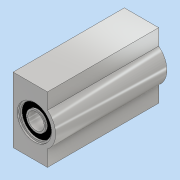
# Autodesk Inventor part: Łożysko liniowe w obudowie SMAG10UU-L
Saved by Autodesk Inventor 2018 (Build 220112000, 112)
## iProperties
Created: 2019-02-01
Part Number: Łożysko liniowe w obudowie SMAG10UU-L
Material: Ogólny
Document SubType Name: Modeling
Designer: Dawid
Density: 1 g/cm^3
Appearance: Aluminium — ciemne
Author: Dawid
Autodesk Inventor part; units mm, degrees
ref_plane "YZ Plane" through (0, 0, 0) normal (1, 0, 0) x (0, 1, 0)
ref_plane "XZ Plane" through (0, 0, 0) normal (0, 1, 0) x (-1, 0, 0)
ref_plane "XY Plane" through (0, 0, 0) normal (0, 0, 1) x (1, 0, 0)
sketch "Szkic1" plane through (0, 0, 0) normal (0, 1, 0) x (-1, 0, 0)
  line L0 (-8, 20) -> (13, 20)
  line L1 (13, 20) -> (13, -20)
  line L2 (13, -20) -> (-8, -20)
  line L3 (-13, 20) -> (13, -20) construction
  line L4 (13, 20) -> (-13, -20) construction
  line L5 (13, 0) -> (0, 0)
  circle A0 centre (0, 0) radius 5
  line L6 (13, 20) -> (-8, 20)
  arc A1 (-8, 10.247) -> (-8, -10.247) centre (0, 0) ccw
  line L7 (-8, 20) -> (-8, 10.247)
  line L8 (-8, -10.247) -> (-8, -20)
  dimension "d0" = 26
  dimension "d1" = 40
  dimension "d2" = 10
  dimension "d3" = 21
  constraints: 18 end point, 5 midpoint, 3 perpendicular, 2 centre point, 2 horizontal, 2 point on circle, 1 parallel
  measures "d0" distance of L1.end L4.end
  measures "d1" distance of L0.end L1.end
  measures "d2" diameter of A0
  measures "d3" distance of L0.start L0.end
extrude "Wyciągnięcie proste1" add sketch "Szkic1" along normal blind 68
sketch "Szkic2" plane through (0, 68, 0) normal (0, 1, 0) x (1, 0, 0)
  circle A0 centre (0, 0) radius 5 projected
  circle A1 centre (0, 0) radius 6
  circle A2 centre (0, 0) radius 10.5
  circle A3 centre (0, 0) radius 9.5
  dimension "d6" = 12
  dimension "d7" = 21
  dimension "d8" = 19
  constraints: 3 centre point, 3 coincident
  measures "d6" diameter of A1
  measures "d7" diameter of A2
  measures "d8" diameter of A3
extrude "Wyciągnięcie proste2" cut sketch "Szkic2" against normal blind 1
sketch "Szkic3" plane through (0, 68, 0) normal (0, 1, 0) x (1, 0, 0)
  circle A0 centre (0, 0) radius 6 projected
  circle A1 centre (0, 0) radius 9.5 projected
extrude "Wyciągnięcie proste3" cut sketch "Szkic3" against normal blind 2
sketch "Szkic4" plane through (0, 0, 0) normal (0, -1, 0) x (1, 0, 0)
  circle A0 centre (0, 0) radius 5
  circle A1 centre (0, 0) radius 6
  circle A2 centre (0, 0) radius 10.5
  circle A3 centre (0, 0) radius 9.5
  dimension "d13" = 12
  dimension "d14" = 21
  dimension "d15" = 19
  constraints: 4 centre point, 3 coincident
  measures "d13" diameter of A1
  measures "d14" diameter of A2
  measures "d15" diameter of A3
extrude "Wyciągnięcie proste4" cut sketch "Szkic4" against normal blind 1
sketch "Szkic5" plane through (0, 0, 0) normal (0, -1, 0) x (1, 0, 0)
  circle A0 centre (0, 0) radius 6 projected
  circle A1 centre (0, 0) radius 9.5 projected
extrude "Wyciągnięcie proste5" cut sketch "Szkic5" against normal blind 2
sketch "Szkic6" plane through (-13, 0, -20) normal (-1, 0, 0) x (0, 0, 1)
  line L0 (0, 0) -> (40, 0) projected
  line L1 (40, 0) -> (40, 68) projected
  line L2 (0, 68) -> (40, 68) projected
  line L3 (0, 0) -> (0, 68) projected
  line L4 (0, 68) -> (20, 68)
  line L5 (20, 68) -> (6, 68)
  line L6 (20, 68) -> (34, 68)
  line L7 (34, 68) -> (34, 0)
  line L8 (0, 0) -> (40, 0) projected
  line L9 (6, 68) -> (6, 0)
  line L10 (34, 68) -> (34, 34)
  line L11 (34, 34) -> (6, 34)
  line L12 (34, 34) -> (34, 57)
  line L13 (34, 57) -> (6, 57)
  line L14 (6, 34) -> (6, 11)
  line L15 (6, 11) -> (34, 11)
  point P0 (20, 0)
  dimension "d20" = 20
  dimension "d21" = 14
  dimension "d22" = 14
  dimension "d23" = 34
  dimension "d24" = 23
  dimension "d25" = 23
  constraints: 22 end point, 8 point on line, 4 perpendicular, 3 midpoint
  measures "d20" distance of L2.start L4.end
  measures "d21" distance of L4.end L5.end
  measures "d22" distance of L4.end L6.end
  measures "d23" distance of L6.end L10.end
  measures "d24" distance of L10.end L12.end
  measures "d25" distance of L11.end L14.end
hole "Otwór1" at (-13, 57, -14) at (-13, 57, 14) at (-13, 11, -14) at (-13, 11, 14) direction (1, 0, 0) diameter 5 depth 12 tip angle 118
thread "Gwint1" size "M5x0.8" class "6H" standard "ANSI Metric M Profile" full length
thread "Gwint2" size "M5x0.8" class "6H" standard "ANSI Metric M Profile" full length
thread "Gwint3" size "M5x0.8" class "6H" standard "ANSI Metric M Profile" full length
thread "Gwint4" size "M5x0.8" class "6H" standard "ANSI Metric M Profile" full length
